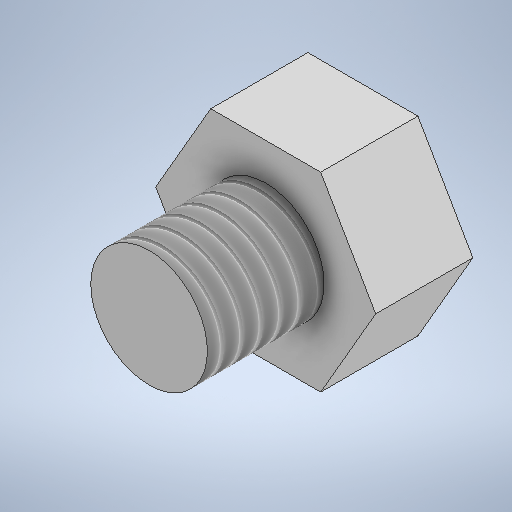
# Autodesk Inventor part: Screw
Saved by Autodesk Inventor 2025.2 (Build 292293000, 293)
## iProperties
Created: 2025-04-06
Part Number: Screw
Material: Generic
Document SubType Name: Modeling
Designer: eason
Density: 1 g/cm^3
Appearance: Default
Author: eason
Autodesk Inventor part; units mm, degrees
ref_plane "YZ Plane" through (0, 0, 0) normal (1, 0, 0) x (0, 1, 0)
ref_plane "XZ Plane" through (0, 0, 0) normal (0, 1, 0) x (-1, 0, 0)
ref_plane "XY Plane" through (0, 0, 0) normal (0, 0, 1) x (1, 0, 0)
sketch "Sketch1" plane through (0, 0, 0) normal (0, 0, 1) x (1, 0, 0)
  circle A0 centre (0, 0) radius 3
  dimension "d0" = 6
  constraints: 1 centre point, 1 coincident
  measures "d0" diameter of A0
extrude "Extrusion1" add sketch "Sketch1" along normal blind 6
sketch "Sketch2" plane through (0, 0, 0) normal (0, 0, 1) x (1, 0, 0)
  circle A0 centre (0, 0) radius 4.9 construction
  line L0 (2.829, 4.9) -> (-2.829, 4.9)
  line L1 (0, -6.86) -> (0, 6.86) projected
  line L2 (-2.829, 4.9) -> (-5.658, 0)
  line L3 (-5.658, 0) -> (-2.829, -4.9)
  line L4 (-2.829, -4.9) -> (2.829, -4.9)
  line L5 (2.829, -4.9) -> (5.658, 0)
  line L6 (5.658, 0) -> (2.829, 4.9)
  point P0 (0, 4.9)
  point P1 (-4.2435, 2.45)
  point P2 (-4.2435, -2.45)
  point P3 (0, -4.9)
  point P4 (4.2435, -2.45)
  point P5 (4.2435, 2.45)
  point P6 (-5.658, 0)
  point P7 (5.658, 0)
  dimension "d3" = 9.8
  dimension "d6" = 360
  constraints: 12 end point, 2 coincident, 1 centre point, 1 horizontal, 1 midpoint, 1 point on line, 1 tangent, 25 other
  measures "d3" diameter of A0
extrude "Extrusion2" add sketch "Sketch2" against normal blind 5
thread "Thread1" size "M6x1" class "6g" standard "ANSI Metric M Profile" full length
body "Solid1"
